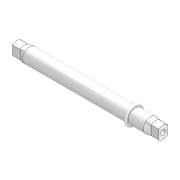
# Autodesk Inventor part: front shaft v3
Saved by Autodesk Inventor 2022 (Build 260153000, 153)
## iProperties
Created: 2024-03-20
Part Number: front shaft v3
Material: Generic
Document SubType Name: Modeling
Designer: david
Density: 1 g/cm^3
Appearance: Smooth - White
Author: david
Autodesk Inventor part; units mm, degrees
ref_plane "YZ Plane" through (0, 0, 0) normal (1, 0, 0) x (0, 1, 0)
ref_plane "XZ Plane" through (0, 0, 0) normal (0, 1, 0) x (-1, 0, 0)
ref_plane "XY Plane" through (0, 0, 0) normal (0, 0, 1) x (1, 0, 0)
sketch "Sketch1" plane through (0, 0, 0) normal (1, 0, 0) x (0, 1, 0)
  circle A0 centre (0, 0) radius 2.85
  dimension "diameter" = 5.7
  constraints: 1 centre point, 1 coincident
  measures "diameter" diameter of A0
extrude "Shaft" add sketch "Sketch1" along normal mid plane 48
ref_plane "Work Plane1" through (26, 0, 0) normal (1, 0, 0) x (0, 0, -1)
sketch "Sketch3" plane through (26, 0, 0) normal (1, 0, 0) x (0, 0, -1)
  circle A0 centre (0, 0) radius 2.85 construction
  circle A1 centre (0, 0) radius 2.5
  line L0 (-1.75, 1.7854) -> (1.75, 1.7854)
  line L1 (1.75, 1.7854) -> (1.75, -1.7854)
  line L2 (1.75, -1.7854) -> (-1.75, -1.7854)
  line L3 (-1.75, -1.7854) -> (-1.75, 1.7854)
  line L4 (-1.75, 1.7854) -> (1.75, -1.7854) construction
  line L5 (1.75, 1.7854) -> (-1.75, -1.7854) construction
  dimension "d77" = 5
  dimension "d76" = 3.5
  constraints: 12 end point, 3 midpoint, 2 coincident, 2 parallel, 1 horizontal, 1 perpendicular, 3 other
  measures "d76" distance of L1.end L2.end
extrude "Wheel Insert Profile" add sketch "Sketch3" along normal blind 3 contours L0 A1 | L1 L2 L3 L0 | A1 L2
loft "Loft1" add section 1 edges at (24, -2.85, 0) section 2 edges at (26, 0, 1.75) (26, 2.5, 0) (26, 0, -1.75) (26, -2.5, 0)
ref_plane "Work Plane2" through (19, 0, 0) normal (-1, 0, 0) x (0, 0, 1)
sketch "Sketch4" plane through (19, 0, 0) normal (-1, 0, 0) x (0, 0, 1)
  circle A0 centre (0, 0) radius 3.75
  dimension "d35" = 7.5
  constraints: 1 centre point, 1 coincident
  measures "d35" diameter of A0
extrude "Stopper" add sketch "Sketch4" against normal blind 1
fillet "Fillet1" radius 0.5 2 edges at (19, 0, -3.75) (20, 0, -3.75)
sketch "Sketch9" plane through (29, 0, 0) normal (1, 0, 0) x (0, 0, -1)
  arc A0 (1.75, 1.7854) -> (-1.75, 1.7854) centre (0, 0) ccw projected
  constraints: 1 coincident
hole "Hole1" at (29, 0, 0) direction (-1, 0, 0) diameter 2 depth 7
mirror "Mirror1" about plane through (0, 0, 0) normal (1, 0, 0) of "Loft1", "Wheel Insert Profile", "Hole1"
body "Solid1"
